2-3-001 Cessna Yoke Grommet_v2 (Autodesk Fusion 360 design; units mm, degrees)
Autodesk Fusion 360 part; units mm, degrees
sketch "Sketch1" plane through (0, 0, 0) normal (0, 0, 1) x (1, 0, 0)
  circle A0 centre (0, 0) radius 18.5511
  arc A1 (-22.4044, 20.933) -> (-29.8061, 7.1934) centre (0, 0) ccw
  line L0 (-21.4764, 21.336) -> (0.0757, 21.336)
  circle A2 centre (-26.2102, 0) radius 5.715
  line L1 (-27.2178, 5.6255) -> (-28.5716, 5.6255)
  arc A3 (-29.8061, 7.1934) -> (-28.5716, 5.6255) centre (-28.5716, 6.8955) ccw
  arc A4 (-21.4764, 21.336) -> (-22.4044, 20.933) centre (-21.4764, 20.066) ccw
  line L2 (0, 0) -> (0, 23.9783) construction
  line L3 (0, 0) -> (-0.8735, 0) construction
  line L4 (-0.8735, 0) -> (-39.1905, 0) construction
  arc A5 (-28.5716, -5.6255) -> (-29.8061, -7.1934) centre (-28.5716, -6.8955) ccw
  circle A6 centre (-26.2102, 0) radius 5.715
  arc A7 (-22.4044, -20.933) -> (-21.4764, -21.336) centre (-21.4764, -20.066) ccw
  line L5 (-21.4764, -21.336) -> (0.0757, -21.336)
  line L6 (-27.2178, -5.6255) -> (-28.5716, -5.6255)
  line L7 (0, 0) -> (-0.8735, 0) construction
  arc A8 (-29.8061, -7.1934) -> (-22.4044, -20.933) centre (0, 0) ccw
  line L8 (0, 0) -> (0.8735, 0) construction
  arc A9 (22.4044, 20.933) -> (21.4764, 21.336) centre (21.4764, 20.066) ccw
  line L9 (0, 0) -> (0.8735, 0) construction
  circle A10 centre (26.2102, 0) radius 5.715
  arc A11 (29.8061, 7.1934) -> (22.4044, 20.933) centre (0, 0) ccw
  line L10 (27.2178, -5.6255) -> (28.5716, -5.6255)
  line L11 (27.2178, 5.6255) -> (28.5716, 5.6255)
  line L12 (21.4764, -21.336) -> (-0.0757, -21.336)
  arc A12 (29.8061, -7.1934) -> (28.5716, -5.6255) centre (28.5716, -6.8955) ccw
  arc A13 (22.4044, -20.933) -> (29.8061, -7.1934) centre (0, 0) ccw
  arc A14 (28.5716, 5.6255) -> (29.8061, 7.1934) centre (28.5716, 6.8955) ccw
  line L13 (21.4764, 21.336) -> (-0.0757, 21.336)
  circle A15 centre (26.2102, 0) radius 5.715
  arc A16 (21.4764, -21.336) -> (22.4044, -20.933) centre (21.4764, -20.066) ccw
  circle A17 centre (-22.86, 14.986) radius 2.159
  circle A18 centre (22.86, 14.986) radius 2.159
  circle A19 centre (22.86, -14.986) radius 2.159
  circle A20 centre (-22.86, -14.986) radius 2.159
  circle A21 centre (0, 0) radius 14.3289
  point P0 (0, 23.9783)
  dimension "d1" = 1.27
  dimension "d2" = 11.43
  dimension "d3" = 4.318
  dimension "d4" = 6.35
  dimension "d5" = 22.86
  dimension "d6" = 21.336
  constraint coincident A0.centre A1.centre
  constraint horizontal L0
  constraint coincident A2 L1.start
  constraint horizontal A0.centre A2.centre
  constraint horizontal L1
  constraint tangent L1 A3
  constraint tangent A1 A3
  constraint tangent A1 A4
  constraint tangent L0 A4
  constraint equal A3 A4
  constraint perpendicular L0 L2
  constraint perpendicular L2 L3
  constraint perpendicular L2 L4
  constraint symmetric A0.centre L4 A1.centre
  constraint symmetric A1 L4 A8
  constraint symmetric L0.end L4 L5.end
  constraint symmetric A2 L4 A6
  constraint symmetric L1.start L4 L6.start
  constraint symmetric L1.end L4 A5.start
  constraint symmetric A1.end L4 A5.end
  constraint symmetric A3 L4 A5
  constraint symmetric L0.start L4 A7.end
  constraint symmetric A1.start L4 A7.start
  constraint symmetric A4 L4 A7
  constraint symmetric L3.end L4 L7.end
  constraint symmetric A0.centre L2 A1.centre
  constraint symmetric A1 L2 A11
  constraint symmetric L0.end L2 L13.end
  constraint symmetric A2 L2 A15
  constraint symmetric L1.start L2 L11.start
  constraint symmetric L1.end L2 L11.end
  constraint symmetric A1.end L2 A11.start
  constraint symmetric A3 L2 A14
  constraint symmetric L0.start L2 A9.end
  constraint symmetric A1.start L2 A9.start
  constraint symmetric A4 L2 A9
  constraint symmetric P0 L2 L2.end
  constraint symmetric L2 A0.centre A1.centre
  constraint symmetric L2 L3.end L8.end
  constraint symmetric L2 L5.end L12.end
  constraint symmetric L2 A7.end L12.start
  constraint symmetric L2 A5.end A12.start
  constraint symmetric L2 A5.start L10.end
  constraint symmetric L2 A7.start A13.start
  constraint symmetric L2 L6.start L10.start
  constraint symmetric L2 A5 A12
  constraint symmetric L2 A6 A10
  constraint symmetric L2 A7 A16
  constraint symmetric L2 A8 A13
  constraint symmetric L2 A17 A18
  constraint symmetric L4 A17 A20
  constraint symmetric L4 A18 A19
  measures "d1" radius of A3
  measures "d2" diameter of A6
  measures "d3" diameter of A17
  measures "d4" distance of L0 A17.centre
  measures "d5" distance of L2 A17.centre
  measures "d6" distance of L0 L4
extrude "Extrude1" add sketch "Sketch1" against normal blind 5.08 contours A0 | A1 L0 A2 L1 A3 A4 A5 A6 A7 L5 L6 A8 A9 A10 A11 L10 L11 L12 A12 A13 A14 L13 A15 A16
ref_plane "WorkPlane1" through (0, 0, 31.75) normal (0, 0, 1) x (1, 0, 0)
sketch "Sketch2" plane through (0, 0, 31.75) normal (0, 0, 1) x (1, 0, 0)
  circle A0 centre (0, 0) radius 16.9336
  circle A1 centre (0, 0) radius 12.7
  dimension "d10" = 25.4
  constraint coincident A0.centre A1.centre
  constraint concentric A0 A1
  measures "d10" diameter of A1
loft "Loft1" add profiles "Sketch1", "Sketch2" section 1 contours A0 section 2
shell "Shell1" thickness 2.54 removed faces 2 at (-4.5896, 0.8413, 31.75) at (-3.49, -1.4237, 0)
extrude "Extrude2" cut 1 faces at (15.3353, -1.5072, 0) along direction (0, 0, -1) blind 27.94
fillet "Fillet1" radius 1.27 1 edges at (-15.7877, 6.1235, 31.75)
fillet "Fillet1" radius 0.635 1 edges at (-13.4165, 5.2038, 31.75)
fillet "Fillet1" radius 1.27 1 edges at (-17.2957, 6.7084, 0)
fillet "Fillet1" radius 2.54 1 edges at (-14.9245, -5.7887, -5.08)
